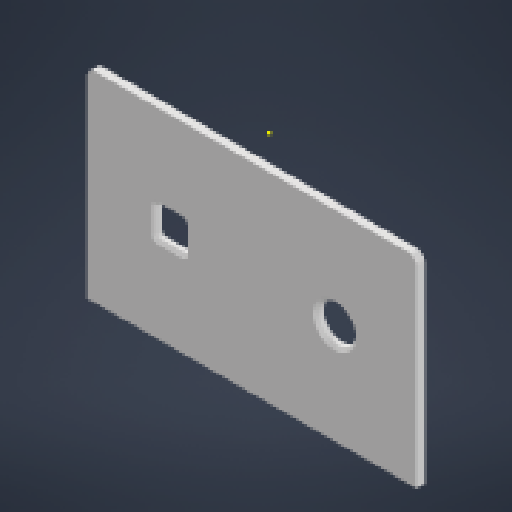
# Autodesk Inventor part: AASTRC Bottom case cover
Saved by Autodesk Inventor 2024.2 (Build 282272000, 272)
## iProperties
Created: 2023-07-16
Part Number: AASTRC Bottom case cover
Material: 일반
Document SubType Name: Modeling
Designer: 6gioc
Density: 1 g/cm^3
Appearance: 기본값
Mass: 130.356 g
Surface Area: 554.511 cm^2
Volume: 130.356 cm^3
Author: 6gioc
## iProperties of the stored document AASTRC Bottom case cover_3D 인쇄.ipt
Created: 2023-11-23
Part Number: AASTRC Bottom case cover_3D 인쇄
Material: 일반
Document SubType Name: Modeling
Designer: 6gioc
Density: 1 g/cm^3
Appearance: 기본값
Author: 6gioc
Autodesk Inventor part; units mm, degrees
ref_plane "YZ Plane" through (0, 0, 0) normal (1, 0, 0) x (0, 1, 0)
ref_plane "XZ Plane" through (0, 0, 0) normal (0, 1, 0) x (-1, 0, 0)
ref_plane "XY Plane" through (0, 0, 0) normal (0, 0, 1) x (1, 0, 0)
sketch "스케치1" plane through (0, 0, 0) normal (0, 0, 1) x (1, 0, 0)
  line L0 (92.7067, -147.2632) -> (-114.2933, -147.2632)
  line L1 (-114.2933, -147.2632) -> (-114.2933, -26.2632)
  line L2 (-109.2933, -21.2632) -> (87.7067, -21.2632)
  line L3 (92.7067, -26.2632) -> (92.7067, -147.2632)
  arc A0 (92.7067, -26.2632) -> (87.7067, -21.2632) centre (87.7067, -26.2632) ccw
  arc A1 (-109.2933, -21.2632) -> (-114.2933, -26.2632) centre (-109.2933, -26.2632) ccw
  point P0 (0, 0)
  point P1 (-114.2933, -21.2632)
  point P2 (92.7067, -21.2632)
  dimension "d0" = 207
  dimension "d1" = 126
  dimension "d10" = 5
  constraints: 8 end point, 4 point on circle, 4 point on line, 4 tangent, 2 centre point, 2 parallel, 1 equal radius, 1 horizontal, 1 perpendicular
  measures "d0" distance of point (-114.293, -21.263) point (92.707, -21.263)
  measures "d1" distance of point (92.707, -21.263) L0.start
  measures "d10" radius of A0
extrude "돌출1" add sketch "스케치1" along normal blind 5
sketch "스케치2" plane through (0, 0, 5) normal (0, 0, 1) x (1, 0, 0)
  point P0 (0, 0)
sketch "스케치4" plane through (0, 0, 5) normal (0, 0, 1) x (1, 0, 0)
  circle A0 centre (40.9567, -84.2632) radius 11.5
  line L0 (-53.0183, -93.7882) -> (-72.0683, -93.7882)
  line L1 (-72.0683, -93.7882) -> (-72.0683, -74.7382)
  line L2 (-72.0683, -74.7382) -> (-53.0183, -74.7382)
  line L3 (-53.0183, -74.7382) -> (-53.0183, -93.7882)
  line L4 (87.7067, -21.2632) -> (-109.2933, -21.2632) projected
  arc A1 (-109.2933, -21.2632) -> (-114.2933, -26.2632) centre (-109.2933, -26.2632) ccw projected
  line L5 (-114.2933, -26.2632) -> (-114.2933, -147.2632) projected
  line L6 (-114.2933, -147.2632) -> (92.7067, -147.2632) projected
  line L7 (92.7067, -147.2632) -> (92.7067, -26.2632) projected
  arc A2 (92.7067, -26.2632) -> (87.7067, -21.2632) centre (87.7067, -26.2632) ccw projected
  point P0 (0, 0)
  point P1 (-62.5433, -93.7882)
  point P2 (-72.0683, -84.2632)
  dimension "d11" = 23
  dimension "d12" = 19.05
  dimension "d13" = 19.05
  dimension "d14" = 53.475
  dimension "d15" = 126
  dimension "d16" = 63
  dimension "d17" = 207
  dimension "d18" = 42.225
  dimension "d19" = 51.75
  constraints: 8 end point, 2 midpoint, 2 parallel, 1 centre point, 1 horizontal, 1 perpendicular
  measures "d11" diameter of A0
  measures "d12" distance of L1.end L2.end
  measures "d13" distance of L0.end L1.end
  measures "d14" distance from line of point (-62.543, -93.788) L6
  measures "d15" distance between parallel lines of L4 L6
  measures "d16" distance from line of A0.centre L6
  measures "d17" distance between parallel lines of L5 L7
  measures "d18" distance from line of L5 point (-72.068, -84.263)
  measures "d19" distance from line of L7 A0.centre
extrude "돌출3" cut sketch "스케치4" against normal blind 10 contours A0 | L0 L1 L2 L3
fillet "모깎기4" radius 2 4 edges at (-53.0183, -93.7882, 2.5) (-72.0683, -93.7882, 2.5) (-53.0183, -74.7382, 2.5) (-72.0683, -74.7382, 2.5)
fillet "모깎기5" radius 4 1 edges at (29.4567, -84.2632, 0) inverted yes
